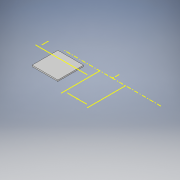
# Autodesk Inventor part: BT002_trajan20_21
Saved by Autodesk Inventor 2022.2 (Build 262287000, 287)
## iProperties
Company: HTBLA Kaindorf
RuleStatus: InUse
Created: 2022-06-07
Part Number: BT002_trajan20_21
Project: Zeichenmaschine_v2
Material: Generisch
Description: GM_Platte
Document SubType Name: Modeling
Designer: trajan20
Density: 1 g/cm^3
Appearance: Vorgabe
Mass: 25.6 g
Surface Area: 140.8 cm^2
Volume: 25.6 cm^3
AfterDocNew0: iProperties-Editor_aufrufen
Author: jan
Keywords: 2021
Autodesk Inventor part; units mm, degrees
ref_plane "YZ Plane" through (0, 0, 0) normal (1, 0, 0) x (0, 1, 0)
ref_plane "XZ Plane" through (0, 0, 0) normal (0, 1, 0) x (-1, 0, 0)
ref_plane "XY Plane" through (0, 0, 0) normal (0, 0, 1) x (1, 0, 0)
derived "MS000_trajan20_21_Zeichenmaschine_Inventor_Masterskizze.ipt"
sketch "Skizze19" plane through (30, -140, -50) normal (1, 0, 0) x (0, 1, 0)
  line L0 (10, -4) -> (-70, -4)
  line L1 (-70, -4) -> (-70, 0)
  line L2 (-70, 0) -> (10, 0)
  line L3 (10, 0) -> (10, -4)
  point P0 (140, 50)
  point P1 (-60, 0)
  point P2 (0, 0)
sketch "Basis" plane through (0, 0, 0) normal (0, 0, 1) x (1, 0, 0)
  line L0 (0, 150) -> (0, -150)
  line L1 (-19.8908, 0) -> (0.1065, 0)
  line L2 (0, -9.9039) -> (0, 9.9039)
  line L3 (30, -50) -> (30, -210)
  line L4 (0, -200) -> (20, -200)
  line L5 (0, -40) -> (120, -40)
  line L6 (0, 40) -> (120, 40)
  line L7 (110, -30) -> (110, 30)
  point P0 (0, 0)
  point P1 (110, 0)
extrude "Extrusion3" add sketch "Skizze19" along normal blind 10 and the other way blind 30
mirror "Spiegeln1" about plane through (0, -170, -52) normal (-1, 0, 0)
equation "\"d5\" = 0.5 * Alu_Prof"
equation "\"d6\" = 0.5 * Bas_Ver_Breite"
equation "\"Alu_Prof\" = 20"
equation "\"Bas_Ver_Breite\" = 60"
